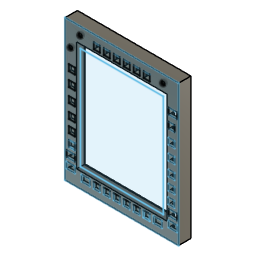
Portrait Iteration 4 v1 (Autodesk Fusion 360 design; units mm, degrees)
Autodesk Fusion 360 part; units mm, degrees
sketch "Sketch1" plane through (0, 0, 0) normal (0, 1, 0) x (1, 0, 0)
  line L0 (-16.7763, -52.2646) -> (91.3257, -52.2646)
  line L1 (91.3257, -52.2646) -> (91.3257, 81.2454)
  line L2 (91.3257, 81.2454) -> (-16.7763, 81.2454)
  line L3 (-16.7763, 81.2454) -> (-16.7763, -52.2646)
  line L4 (-36.7763, -77.2646) -> (111.3257, -77.2646)
  line L5 (111.3257, -77.2646) -> (111.3257, 106.2454)
  line L6 (111.3257, 106.2454) -> (-36.7763, 106.2454)
  line L7 (-36.7763, 106.2454) -> (-36.7763, -77.2646)
  dimension "d1" = 108.102
  dimension "d2" = 133.51
  dimension "d3" = 20
  dimension "d4" = 25
  dimension "d5" = 20
  dimension "d6" = 25
  constraint horizontal L0
  constraint vertical L1
  constraint horizontal L2
  constraint vertical L3
  constraint horizontal L4
  constraint vertical L5
  constraint horizontal L6
  constraint vertical L7
  measures "d1" distance of L0.start L0.end
  measures "d2" distance of L0.start L2.end
  measures "d3" distance of L1 L5
  measures "d4" distance of L2 L6
  measures "d5" distance of L3 L7
  measures "d6" distance of L0 L4
extrude "Extrude1" add sketch "Sketch1" along normal blind 16
chamfer "Chamfer1" distance 5 angle 45 4 edges at (-16.7763, 0, -14.4904) (37.2747, 0, 52.2646) (91.3257, 0, -14.4904) (37.2747, 0, -81.2454)
sketch "Sketch2" plane through (0, 0, 0) normal (0, -1, 0) x (1, 0, 0)
  line L0 (-36.7763, 77.2646) -> (-36.7763, -106.2454)
  line L1 (-36.7763, -106.2454) -> (111.3257, -106.2454)
  line L2 (111.3257, -106.2454) -> (111.3257, 77.2646)
  line L3 (111.3257, 77.2646) -> (-36.7763, 77.2646)
  line L4 (-21.7763, -86.2454) -> (-21.7763, 57.2646)
  line L5 (-21.7763, 57.2646) -> (96.3257, 57.2646)
  line L6 (96.3257, 57.2646) -> (96.3257, -86.2454)
  line L7 (96.3257, -86.2454) -> (-21.7763, -86.2454)
  line L8 (-31.7763, 27.2646) -> (-23.7763, 27.2646)
  line L9 (-23.7763, 27.2646) -> (-23.7763, 19.2646)
  line L10 (-23.7763, 19.2646) -> (-31.7763, 19.2646)
  line L11 (-31.7763, 19.2646) -> (-31.7763, 27.2646)
  line L12 (-31.7763, -8.7354) -> (-23.7763, -8.7354)
  line L13 (-23.7763, -8.7354) -> (-23.7763, -16.7354)
  line L14 (-23.7763, -16.7354) -> (-31.7763, -16.7354)
  line L15 (-31.7763, -16.7354) -> (-31.7763, -8.7354)
  line L16 (-31.7763, 9.2646) -> (-23.7763, 9.2646)
  line L17 (-23.7763, 9.2646) -> (-23.7763, 1.2646)
  line L18 (-23.7763, 1.2646) -> (-31.7763, 1.2646)
  line L19 (-31.7763, 1.2646) -> (-31.7763, 9.2646)
  line L20 (-31.7763, -26.7354) -> (-23.7763, -26.7354)
  line L21 (-23.7763, -26.7354) -> (-23.7763, -34.7354)
  line L22 (-23.7763, -34.7354) -> (-31.7763, -34.7354)
  line L23 (-31.7763, -34.7354) -> (-31.7763, -26.7354)
  line L24 (-31.7763, -42.7354) -> (-23.7763, -42.7354)
  line L25 (-23.7763, -42.7354) -> (-23.7763, -50.7354)
  line L26 (-23.7763, -50.7354) -> (-31.7763, -50.7354)
  line L27 (-31.7763, -50.7354) -> (-31.7763, -42.7354)
  line L28 (-31.7763, -58.2454) -> (-23.7763, -58.2454)
  line L29 (-23.7763, -58.2454) -> (-23.7763, -66.2454)
  line L30 (-23.7763, -66.2454) -> (-31.7763, -66.2454)
  line L31 (-31.7763, -66.2454) -> (-31.7763, -58.2454)
  line L32 (0.7237, 68.2646) -> (8.7237, 68.2646)
  line L33 (8.7237, 68.2646) -> (8.7237, 60.2646)
  line L34 (8.7237, 60.2646) -> (0.7237, 60.2646)
  line L35 (0.7237, 60.2646) -> (0.7237, 68.2646)
  line L36 (13.7237, 60.2646) -> (13.7237, 68.2646)
  line L37 (13.7237, 68.2646) -> (21.7237, 68.2646)
  line L38 (21.7237, 68.2646) -> (21.7237, 60.2646)
  line L39 (21.7237, 60.2646) -> (13.7237, 60.2646)
  line L40 (26.7237, 60.2646) -> (26.7237, 68.2646)
  line L41 (26.7237, 68.2646) -> (34.7237, 68.2646)
  line L42 (34.7237, 68.2646) -> (34.7237, 60.2646)
  line L43 (34.7237, 60.2646) -> (26.7237, 60.2646)
  line L44 (65.7237, 60.2646) -> (65.7237, 68.2646)
  line L45 (65.7237, 68.2646) -> (73.7237, 68.2646)
  line L46 (73.7237, 68.2646) -> (73.7237, 60.2646)
  line L47 (73.7237, 60.2646) -> (65.7237, 60.2646)
  line L48 (39.7237, 60.2646) -> (39.7237, 68.2646)
  line L49 (39.7237, 68.2646) -> (47.7237, 68.2646)
  line L50 (47.7237, 68.2646) -> (47.7237, 60.2646)
  line L51 (47.7237, 60.2646) -> (39.7237, 60.2646)
  line L52 (52.7237, 60.2646) -> (52.7237, 68.2646)
  line L53 (52.7237, 68.2646) -> (60.7237, 68.2646)
  line L54 (60.7237, 68.2646) -> (60.7237, 60.2646)
  line L55 (60.7237, 60.2646) -> (52.7237, 60.2646)
  line L56 (98.3257, 27.2646) -> (106.3257, 27.2646)
  line L57 (106.3257, 27.2646) -> (106.3257, 19.2646)
  line L58 (106.3257, 19.2646) -> (98.3257, 19.2646)
  line L59 (98.3257, 19.2646) -> (98.3257, 27.2646)
  line L60 (98.3257, 9.2646) -> (106.3257, 9.2646)
  line L61 (106.3257, 9.2646) -> (106.3257, 1.2646)
  line L62 (106.3257, 1.2646) -> (98.3257, 1.2646)
  line L63 (98.3257, 1.2646) -> (98.3257, 9.2646)
  line L64 (98.3257, -8.7354) -> (106.3257, -8.7354)
  line L65 (106.3257, -8.7354) -> (106.3257, -16.7354)
  line L66 (106.3257, -16.7354) -> (98.3257, -16.7354)
  line L67 (98.3257, -16.7354) -> (98.3257, -8.7354)
  line L68 (98.3257, -26.7354) -> (106.3257, -26.7354)
  line L69 (106.3257, -26.7354) -> (106.3257, -34.7354)
  line L70 (106.3257, -34.7354) -> (98.3257, -34.7354)
  line L71 (98.3257, -34.7354) -> (98.3257, -26.7354)
  line L72 (98.3257, -42.7354) -> (106.3257, -42.7354)
  line L73 (106.3257, -42.7354) -> (106.3257, -50.7354)
  line L74 (106.3257, -50.7354) -> (98.3257, -50.7354)
  line L75 (98.3257, -50.7354) -> (98.3257, -42.7354)
  line L76 (97.8961, -58.2454) -> (105.8961, -58.2454)
  line L77 (105.8961, -58.2454) -> (105.8961, -66.2454)
  line L78 (105.8961, -66.2454) -> (97.8961, -66.2454)
  line L79 (97.8961, -66.2454) -> (97.8961, -58.2454)
  line L80 (0.7237, -89.2454) -> (8.7237, -89.2454)
  line L81 (8.7237, -89.2454) -> (8.7237, -97.2454)
  line L82 (8.7237, -97.2454) -> (0.7237, -97.2454)
  line L83 (0.7237, -97.2454) -> (0.7237, -89.2454)
  line L84 (13.7237, -89.2454) -> (21.7237, -89.2454)
  line L85 (21.7237, -89.2454) -> (21.7237, -97.2454)
  line L86 (13.7237, -97.2454) -> (13.7237, -89.2454)
  line L87 (21.7237, -97.2454) -> (13.7237, -97.2454)
  line L88 (26.7237, -89.2454) -> (34.7237, -89.2454)
  line L89 (34.7237, -89.2454) -> (34.7237, -97.2454)
  line L90 (26.7237, -97.2454) -> (26.7237, -89.2454)
  line L91 (34.7237, -97.2454) -> (26.7237, -97.2454)
  line L92 (39.7237, -89.2454) -> (47.7237, -89.2454)
  line L93 (47.7237, -89.2454) -> (47.7237, -97.2454)
  line L94 (39.7237, -97.2454) -> (39.7237, -89.2454)
  line L95 (47.7237, -97.2454) -> (39.7237, -97.2454)
  line L96 (52.7237, -89.2454) -> (60.7237, -89.2454)
  line L97 (60.7237, -89.2454) -> (60.7237, -97.2454)
  line L98 (52.7237, -97.2454) -> (52.7237, -89.2454)
  line L99 (60.7237, -97.2454) -> (52.7237, -97.2454)
  line L100 (65.7237, -89.2454) -> (73.7237, -89.2454)
  line L101 (73.7237, -89.2454) -> (73.7237, -97.2454)
  line L102 (65.7237, -97.2454) -> (65.7237, -89.2454)
  line L103 (73.7237, -97.2454) -> (65.7237, -97.2454)
  line L104 (65.7237, -97.2454) -> (65.7237, -89.2454)
  line L105 (65.7237, -89.2454) -> (73.7237, -89.2454)
  line L106 (73.7237, -89.2454) -> (73.7237, -97.2454)
  line L107 (73.7237, -97.2454) -> (65.7237, -97.2454)
  line L108 (78.7237, -97.2454) -> (78.7237, -89.2454)
  line L109 (78.7237, -89.2454) -> (89.7237, -89.2454)
  line L110 (89.7237, -89.2454) -> (89.7237, -97.2454)
  line L111 (89.7237, -97.2454) -> (78.7237, -97.2454)
  line L112 (-15.2763, -89.2454) -> (-4.2763, -89.2454)
  line L113 (-4.2763, -89.2454) -> (-4.2763, -97.2454)
  line L114 (-4.2763, -97.2454) -> (-15.2763, -97.2454)
  line L115 (-15.2763, -97.2454) -> (-15.2763, -89.2454)
  line L116 (-31.7763, -58.2454) -> (-23.7763, -58.2454)
  line L117 (-23.7763, -58.2454) -> (-23.7763, -66.2454)
  line L118 (-23.7763, -66.2454) -> (-31.7763, -66.2454)
  line L119 (-31.7763, -66.2454) -> (-31.7763, -58.2454)
  line L120 (-34.7763, -71.2454) -> (-23.7763, -71.2454)
  line L121 (-23.7763, -71.2454) -> (-23.7763, -79.2454)
  line L122 (-23.7763, -79.2454) -> (-34.7763, -79.2454)
  line L123 (-34.7763, -79.2454) -> (-34.7763, -71.2454)
  line L124 (-34.7763, -84.2454) -> (-23.7763, -84.2454)
  line L125 (-23.7763, -84.2454) -> (-23.7763, -92.2454)
  line L126 (-23.7763, -92.2454) -> (-34.7763, -92.2454)
  line L127 (-34.7763, -92.2454) -> (-34.7763, -84.2454)
  line L128 (98.3257, 43.2646) -> (109.3257, 43.2646)
  line L129 (109.3257, 43.2646) -> (109.3257, 35.2646)
  line L130 (109.3257, 35.2646) -> (98.3257, 35.2646)
  line L131 (98.3257, 35.2646) -> (98.3257, 43.2646)
  line L132 (98.3257, -71.2454) -> (109.3257, -71.2454)
  line L133 (109.3257, -71.2454) -> (109.3257, -79.2454)
  line L134 (109.3257, -79.2454) -> (98.3257, -79.2454)
  line L135 (98.3257, -79.2454) -> (98.3257, -71.2454)
  line L136 (98.3257, -84.2454) -> (109.3257, -84.2454)
  line L137 (109.3257, -84.2454) -> (109.3257, -92.2454)
  line L138 (109.3257, -92.2454) -> (98.3257, -92.2454)
  line L139 (98.3257, -92.2454) -> (98.3257, -84.2454)
  circle A0 centre (-16.7763, 67.2646) radius 1.8
  circle A1 centre (91.3257, 67.2646) radius 1.8
  circle A2 centre (-29.2763, 47.2646) radius 1.8
  dimension "d10" = 8
  dimension "d11" = 8
  dimension "d12" = 8
  dimension "d13" = 8
  dimension "d14" = 8
  dimension "d15" = 8
  dimension "d16" = 8
  dimension "d17" = 8
  dimension "d18" = 8
  dimension "d19" = 8
  dimension "d20" = 8
  dimension "d21" = 8
  dimension "d22" = 8
  dimension "d24" = 8
  dimension "d26" = 8
  dimension "d28" = 8
  dimension "d30" = 8
  dimension "d32" = 8
  dimension "d34" = 148.102
  dimension "d35" = 50
  dimension "d36" = 2
  dimension "d37" = 2
  dimension "d38" = 68
  dimension "d39" = 86
  dimension "d40" = 2
  dimension "d41" = 2
  dimension "d42" = 2
  dimension "d43" = 2
  dimension "d44" = 104
  dimension "d45" = 120
  dimension "d47" = 3
  dimension "d48" = 3
  dimension "d49" = 3
  dimension "d50" = 3
  dimension "d51" = 3
  dimension "d52" = 3
  dimension "d53" = 37.5
  dimension "d54" = 50.5
  dimension "d57" = 76.5
  dimension "d58" = 89.5
  dimension "d59" = 63.5
  dimension "d60" = 102.5
  dimension "d61" = 5
  dimension "d62" = 5
  dimension "d63" = 5
  dimension "d64" = 5
  dimension "d65" = 5
  dimension "d66" = 37.602
  dimension "d67" = 37.5
  dimension "d70" = 8
  dimension "d71" = 10
  dimension "d73" = 8
  dimension "d74" = 8
  dimension "d75" = 2
  dimension "d76" = 8
  dimension "d77" = 8
  dimension "d78" = 8
  dimension "d79" = 8
  dimension "d80" = 8
  dimension "d81" = 8
  dimension "d82" = 8
  dimension "d83" = 8
  dimension "d84" = 8
  dimension "d85" = 8
  dimension "d86" = 8
  dimension "d87" = 8
  dimension "d88" = 8
  dimension "d89" = 8
  dimension "d90" = 8
  dimension "d91" = 8
  dimension "d92" = 8
  dimension "d93" = 5
  dimension "d94" = 5
  dimension "d95" = 5
  dimension "d96" = 5
  dimension "d97" = 5
  dimension "d98" = 3
  dimension "d99" = 3
  dimension "d100" = 3
  dimension "d101" = 8
  dimension "d102" = 8
  dimension "d103" = 3
  dimension "d104" = 3
  dimension "d105" = 3
  dimension "d106" = 8
  dimension "d107" = 11
  dimension "d108" = 5
  dimension "d109" = 11
  dimension "d110" = 5
  dimension "d111" = 8
  dimension "d112" = 8
  dimension "d113" = 11
  dimension "d114" = 8
  dimension "d115" = 2
  dimension "d116" = 5
  dimension "d117" = 11
  dimension "d118" = 8
  dimension "d119" = 5
  dimension "d120" = 11
  dimension "d121" = 8
  dimension "d122" = 2
  dimension "d123" = 8
  dimension "d124" = 11
  dimension "d125" = 8
  dimension "d126" = 11
  dimension "d127" = 5
  dimension "d128" = 2
  dimension "d129" = 11
  dimension "d130" = 8
  dimension "d131" = 11
  dimension "d132" = 5
  dimension "d133" = 3.6
  dimension "d134" = 10
  dimension "d135" = 20
  dimension "d136" = 37.5
  dimension "d137" = 20
  dimension "d138" = 3.6
  dimension "d139" = 10
  dimension "d140" = 20
  dimension "d141" = 3.6
  dimension "d142" = 5
  dimension "d143" = 7.5
  dimension "d144" = 7.5
  dimension "d145" = 30
  constraint horizontal L8
  constraint vertical L9
  constraint horizontal L10
  constraint vertical L11
  constraint horizontal L12
  constraint vertical L13
  constraint horizontal L14
  constraint vertical L15
  constraint horizontal L16
  constraint vertical L17
  constraint horizontal L18
  constraint vertical L19
  constraint horizontal L20
  constraint vertical L21
  constraint horizontal L22
  constraint vertical L23
  constraint horizontal L24
  constraint vertical L25
  constraint horizontal L26
  constraint vertical L27
  constraint horizontal L28
  constraint vertical L29
  constraint horizontal L30
  constraint vertical L31
  constraint horizontal L32
  constraint vertical L33
  constraint horizontal L34
  constraint vertical L35
  constraint horizontal L37
  constraint vertical L38
  constraint horizontal L39
  constraint vertical L36
  constraint horizontal L41
  constraint vertical L42
  constraint horizontal L43
  constraint vertical L40
  constraint horizontal L45
  constraint vertical L46
  constraint horizontal L47
  constraint vertical L44
  constraint horizontal L49
  constraint vertical L50
  constraint horizontal L51
  constraint vertical L48
  constraint horizontal L53
  constraint vertical L54
  constraint horizontal L55
  constraint vertical L52
  constraint horizontal L56
  constraint vertical L57
  constraint horizontal L58
  constraint vertical L59
  constraint horizontal L60
  constraint vertical L61
  constraint horizontal L62
  constraint vertical L63
  constraint horizontal L64
  constraint vertical L65
  constraint horizontal L66
  constraint vertical L67
  constraint horizontal L68
  constraint vertical L69
  constraint horizontal L70
  constraint vertical L71
  constraint horizontal L72
  constraint vertical L73
  constraint horizontal L74
  constraint vertical L75
  constraint horizontal L76
  constraint vertical L77
  constraint horizontal L78
  constraint vertical L79
  constraint horizontal L80
  constraint vertical L81
  constraint horizontal L82
  constraint vertical L83
  constraint horizontal L84
  constraint vertical L85
  constraint horizontal L87
  constraint vertical L86
  constraint horizontal L88
  constraint vertical L89
  constraint horizontal L91
  constraint vertical L90
  constraint horizontal L100
  constraint vertical L101
  constraint horizontal L103
  constraint vertical L102
  constraint horizontal L92
  constraint vertical L93
  constraint horizontal L95
  constraint vertical L94
  constraint horizontal L96
  constraint vertical L97
  constraint horizontal L99
  constraint vertical L98
  constraint horizontal L105
  constraint vertical L106
  constraint horizontal L107
  constraint vertical L104
  constraint horizontal L109
  constraint vertical L110
  constraint horizontal L111
  constraint vertical L108
  constraint horizontal L112
  constraint vertical L113
  constraint horizontal L114
  constraint vertical L115
  constraint horizontal L116
  constraint vertical L117
  constraint horizontal L118
  constraint vertical L119
  constraint horizontal L120
  constraint vertical L121
  constraint horizontal L122
  constraint vertical L123
  constraint horizontal L124
  constraint vertical L125
  constraint horizontal L126
  constraint vertical L127
  constraint horizontal L128
  constraint vertical L129
  constraint horizontal L130
  constraint vertical L131
  constraint horizontal L132
  constraint vertical L133
  constraint horizontal L134
  constraint vertical L135
  constraint horizontal L136
  constraint vertical L137
  constraint horizontal L138
  constraint vertical L139
  measures "d10" distance of L8.start L8.end
  measures "d11" distance of L8.start L10.end
  measures "d12" distance of L12.end L12.start
  measures "d13" distance of L14.end L12.start
  measures "d14" distance of L16.end L16.start
  measures "d15" distance of L18.end L16.start
  measures "d16" distance of L20.end L20.start
  measures "d17" distance of L22.end L20.start
  measures "d18" distance of L24.end L24.start
  measures "d19" distance of L26.end L24.start
  measures "d20" distance of L28.end L28.start
  measures "d21" distance of L30.end L28.start
  measures "d22" distance of L32.end L32.start
  measures "d24" distance of L37.end L36.end
  measures "d26" distance of L41.end L40.end
  measures "d28" distance of L45.end L44.end
  measures "d30" distance of L49.end L48.end
  measures "d32" distance of L53.end L52.end
  measures "d34" distance of L0.start L2.end
  measures "d35" distance of L3 L8
  measures "d36" distance of L4 L9
  measures "d37" distance of L4 L17
  measures "d38" distance of L3 L16
  measures "d39" distance of L3 L12
  measures "d40" distance of L4 L13
  measures "d41" distance of L4 L21
  measures "d42" distance of L4 L25
  measures "d43" distance of L4 L29
  measures "d44" distance of L3 L20
  measures "d45" distance of L3 L24
  measures "d47" distance of L5 L34
  measures "d48" distance of L5 L39
  measures "d49" distance of L5 L43
  measures "d50" distance of L5 L47
  measures "d51" distance of L5 L51
  measures "d52" distance of L5 L55
  measures "d53" distance of L0 L35
  measures "d54" distance of L0 L36
  measures "d57" distance of L0 L48
  measures "d58" distance of L0 L52
  measures "d59" distance of L0 L40
  measures "d60" distance of L0 L44
  measures "d61" distance of L33 L36
  measures "d62" distance of L38 L40
  measures "d63" distance of L42 L48
  measures "d64" distance of L50 L52
  measures "d65" distance of L44 L54
  measures "d66" distance of L2 L46
  measures "d67" distance of L0 L35
  measures "d70" distance of L16.end L16.start
  measures "d71" distance of L10 L16
  measures "d73" distance of L56.end L56.start
  measures "d74" distance of L58.end L56.start
  measures "d75" distance of L6 L59
  measures "d76" distance of L60.start L60.end
  measures "d77" distance of L60.start L62.end
  measures "d78" distance of L60.start L60.end
  measures "d79" distance of L64.start L64.end
  measures "d80" distance of L64.start L66.end
  measures "d81" distance of L68.end L68.start
  measures "d82" distance of L68.start L70.end
  measures "d83" distance of L72.end L72.start
  measures "d84" distance of L72.start L74.end
  measures "d85" distance of L76.start L76.end
  measures "d86" distance of L78.end L76.start
  measures "d87" distance of L80.end L80.start
  measures "d88" distance of L84.start L84.end
  measures "d89" distance of L88.start L88.end
  measures "d90" distance of L100.end L100.start
  measures "d91" distance of L92.start L92.end
  measures "d92" distance of L96.end L96.start
  measures "d93" distance of L81 L86
  measures "d94" distance of L85 L90
  measures "d95" distance of L89 L94
  measures "d96" distance of L93 L98
  measures "d97" distance of L97 L102
  measures "d98" distance of L7 L80
  measures "d99" distance of L7 L84
  measures "d100" distance of L7 L88
  measures "d101" distance of L92.start L92.end
  measures "d102" distance of L92.start L92.end
  measures "d103" distance of L7 L92
  measures "d104" distance of L7 L96
  measures "d105" distance of L7 L100
  measures "d106" distance of L100.end L100.start
  measures "d107" distance of L108.end L109.end
  measures "d108" distance of L106 L108
  measures "d109" distance of L112.start L112.end
  measures "d110" distance of L83 L113
  measures "d111" distance of L28.start L28.end
  measures "d112" distance of L30.end L28.start
  measures "d113" distance of L120.start L120.end
  measures "d114" distance of L120.start L122.end
  measures "d115" distance of L4 L121
  measures "d116" distance of L118 L120
  measures "d117" distance of L124.end L124.start
  measures "d118" distance of L126.end L124.start
  measures "d119" distance of L122 L124
  measures "d120" distance of L128.start L128.end
  measures "d121" distance of L128.start L130.end
  measures "d122" distance of L6 L131
  measures "d123" distance of L56 L130
  measures "d124" distance of L132.start L132.end
  measures "d125" distance of L132.start L134.end
  measures "d126" distance of L132.start L132.end
  measures "d127" distance of L78 L132
  measures "d128" distance of L6 L135
  measures "d129" distance of L136.end L136.start
  measures "d130" distance of L136.start L138.end
  measures "d131" distance of L136.end L136.start
  measures "d132" distance of L134 L136
  measures "d133" diameter of A0
  measures "d134" distance of L3 A0.centre
  measures "d135" distance of L3 L5
  measures "d136" distance of L0 L35
  measures "d137" distance of L0 A0.centre
  measures "d138" diameter of A1
  measures "d139" distance of L3 A1.centre
  measures "d140" distance of L2 A1.centre
  measures "d141" diameter of A2
  measures "d142" distance of L0 L11
  measures "d143" distance of L0 A2.centre
  measures "d144" distance of L4 A2.centre
  measures "d145" distance of L3 A2.centre
extrude "Extrude2" cut sketch "Sketch2" against normal through all contours L8 L9 L10 L11 | L12 L13 L14 L15 | L16 L17 L18 L19 | L20 L21 L22 L23 | L24 L25 L26 L27 | L28 L29 L30 L31 L116 L117 L118 L119 | L32 L33 L34 L35 | L36 L37 L38 L39 | L40 L41 L42 L43 | L44 L45 L46 L47 | L48 L49 L50 L51 | L52 L53 L54 L55 | L56 L57 L58 L59 | L60 L61 L62 L63 | L64 L65 L66 L67 | L68 L69 L70 L71 | L72 L73 L74 L75 | L76 L77 L78 L79 | L80 L81 L82 L83 | L84 L85 L86 L87 | L88 L89 L90 L91 | L92 L93 L94 L95 | L96 L97 L98 L99 | L100 L101 L102 L103 L104 L105 L106 L107 | L108 L109 L110 L111 | L112 L113 L114 L115 | L120 L121 L122 L123 | L124 L125 L126 L127 | L128 L129 L130 L131 | L132 L133 L134 L135 | L136 L137 L138 L139 | A0 | A2
extrude "Extrude3" cut sketch "Sketch2" against normal through all contours A1
sketch "Sketch3" plane through (0, 16, 0) normal (0, 1, 0) x (-1, 0, 0)
  circle A0 centre (-91.3257, 67.2646) radius 1.8
  line L0 (34.7763, -71.2454) -> (34.7763, -79.2454)
  line L1 (34.7763, -79.2454) -> (23.7763, -79.2454)
  line L2 (23.7763, -79.2454) -> (23.7763, -71.2454)
  line L3 (23.7763, -71.2454) -> (34.7763, -71.2454)
  line L4 (-13.7237, -97.2454) -> (-21.7237, -97.2454)
  line L5 (-21.7237, -97.2454) -> (-21.7237, -89.2454)
  line L6 (-21.7237, -89.2454) -> (-13.7237, -89.2454)
  line L7 (-13.7237, -89.2454) -> (-13.7237, -97.2454)
  line L8 (-65.7237, -97.2454) -> (-73.7237, -97.2454)
  line L9 (-73.7237, -97.2454) -> (-73.7237, -89.2454)
  line L10 (-73.7237, -89.2454) -> (-65.7237, -89.2454)
  line L11 (-65.7237, -89.2454) -> (-65.7237, -97.2454)
  line L12 (-97.8961, -58.2454) -> (-97.8961, -66.2454)
  line L13 (-97.8961, -66.2454) -> (-105.8961, -66.2454)
  line L14 (-105.8961, -66.2454) -> (-105.8961, -58.2454)
  line L15 (-105.8961, -58.2454) -> (-97.8961, -58.2454)
  line L16 (-98.3257, 9.2646) -> (-98.3257, 1.2646)
  line L17 (-98.3257, 1.2646) -> (-106.3257, 1.2646)
  line L18 (-106.3257, 1.2646) -> (-106.3257, 9.2646)
  line L19 (-106.3257, 9.2646) -> (-98.3257, 9.2646)
  line L20 (-52.7237, 60.2646) -> (-60.7237, 60.2646)
  line L21 (-60.7237, 60.2646) -> (-60.7237, 68.2646)
  line L22 (-60.7237, 68.2646) -> (-52.7237, 68.2646)
  line L23 (-52.7237, 68.2646) -> (-52.7237, 60.2646)
  line L24 (-0.7237, 68.2646) -> (-0.7237, 60.2646)
  line L25 (-0.7237, 60.2646) -> (-8.7237, 60.2646)
  line L26 (-8.7237, 60.2646) -> (-8.7237, 68.2646)
  line L27 (-8.7237, 68.2646) -> (-0.7237, 68.2646)
  line L28 (31.7763, -8.7354) -> (31.7763, -16.7354)
  line L29 (31.7763, -16.7354) -> (23.7763, -16.7354)
  line L30 (23.7763, -16.7354) -> (23.7763, -8.7354)
  line L31 (23.7763, -8.7354) -> (31.7763, -8.7354)
  line L32 (31.7763, 9.2646) -> (31.7763, 1.2646)
  line L33 (31.7763, 1.2646) -> (23.7763, 1.2646)
  line L34 (23.7763, 1.2646) -> (23.7763, 9.2646)
  line L35 (23.7763, 9.2646) -> (31.7763, 9.2646)
  circle A1 centre (16.7763, 67.2646) radius 1.8
  line L36 (-39.7237, 60.2646) -> (-47.7237, 60.2646)
  line L37 (-47.7237, 60.2646) -> (-47.7237, 68.2646)
  line L38 (-47.7237, 68.2646) -> (-39.7237, 68.2646)
  line L39 (-39.7237, 68.2646) -> (-39.7237, 60.2646)
  line L40 (-98.3257, 27.2646) -> (-98.3257, 19.2646)
  line L41 (-98.3257, 19.2646) -> (-106.3257, 19.2646)
  line L42 (-106.3257, 19.2646) -> (-106.3257, 27.2646)
  line L43 (-106.3257, 27.2646) -> (-98.3257, 27.2646)
  line L44 (-98.3257, -42.7354) -> (-98.3257, -50.7354)
  line L45 (-98.3257, -50.7354) -> (-106.3257, -50.7354)
  line L46 (-106.3257, -50.7354) -> (-106.3257, -42.7354)
  line L47 (-106.3257, -42.7354) -> (-98.3257, -42.7354)
  line L48 (-78.7237, -97.2454) -> (-89.7237, -97.2454)
  line L49 (-89.7237, -97.2454) -> (-89.7237, -89.2454)
  line L50 (-89.7237, -89.2454) -> (-78.7237, -89.2454)
  line L51 (-78.7237, -89.2454) -> (-78.7237, -97.2454)
  line L52 (-26.7237, -97.2454) -> (-34.7237, -97.2454)
  line L53 (-34.7237, -97.2454) -> (-34.7237, -89.2454)
  line L54 (-34.7237, -89.2454) -> (-26.7237, -89.2454)
  line L55 (-26.7237, -89.2454) -> (-26.7237, -97.2454)
  line L56 (34.7763, -84.2454) -> (34.7763, -92.2454)
  line L57 (34.7763, -92.2454) -> (23.7763, -92.2454)
  line L58 (23.7763, -92.2454) -> (23.7763, -84.2454)
  line L59 (23.7763, -84.2454) -> (34.7763, -84.2454)
  line L60 (31.7763, -58.2454) -> (31.7763, -66.2454)
  line L61 (31.7763, -66.2454) -> (23.7763, -66.2454)
  line L62 (23.7763, -66.2454) -> (23.7763, -58.2454)
  line L63 (23.7763, -58.2454) -> (31.7763, -58.2454)
  line L64 (-0.7237, -89.2454) -> (-0.7237, -97.2454)
  line L65 (-0.7237, -97.2454) -> (-8.7237, -97.2454)
  line L66 (-8.7237, -97.2454) -> (-8.7237, -89.2454)
  line L67 (-8.7237, -89.2454) -> (-0.7237, -89.2454)
  line L68 (-52.7237, -97.2454) -> (-60.7237, -97.2454)
  line L69 (-60.7237, -97.2454) -> (-60.7237, -89.2454)
  line L70 (-60.7237, -89.2454) -> (-52.7237, -89.2454)
  line L71 (-52.7237, -89.2454) -> (-52.7237, -97.2454)
  line L72 (-98.3257, -71.2454) -> (-98.3257, -79.2454)
  line L73 (-98.3257, -79.2454) -> (-109.3257, -79.2454)
  line L74 (-109.3257, -79.2454) -> (-109.3257, -71.2454)
  line L75 (-109.3257, -71.2454) -> (-98.3257, -71.2454)
  line L76 (-98.3257, -8.7354) -> (-98.3257, -16.7354)
  line L77 (-98.3257, -16.7354) -> (-106.3257, -16.7354)
  line L78 (-106.3257, -16.7354) -> (-106.3257, -8.7354)
  line L79 (-106.3257, -8.7354) -> (-98.3257, -8.7354)
  line L80 (-65.7237, 60.2646) -> (-73.7237, 60.2646)
  line L81 (-73.7237, 60.2646) -> (-73.7237, 68.2646)
  line L82 (-73.7237, 68.2646) -> (-65.7237, 68.2646)
  line L83 (-65.7237, 68.2646) -> (-65.7237, 60.2646)
  line L84 (-13.7237, 60.2646) -> (-21.7237, 60.2646)
  line L85 (-21.7237, 60.2646) -> (-21.7237, 68.2646)
  line L86 (-21.7237, 68.2646) -> (-13.7237, 68.2646)
  line L87 (-13.7237, 68.2646) -> (-13.7237, 60.2646)
  line L88 (31.7763, -26.7354) -> (31.7763, -34.7354)
  line L89 (31.7763, -34.7354) -> (23.7763, -34.7354)
  line L90 (23.7763, -34.7354) -> (23.7763, -26.7354)
  line L91 (23.7763, -26.7354) -> (31.7763, -26.7354)
  line L92 (31.7763, 27.2646) -> (31.7763, 19.2646)
  line L93 (31.7763, 19.2646) -> (23.7763, 19.2646)
  line L94 (23.7763, 19.2646) -> (23.7763, 27.2646)
  line L95 (23.7763, 27.2646) -> (31.7763, 27.2646)
  circle A2 centre (29.2763, 47.2646) radius 1.8
  line L96 (-26.7237, 60.2646) -> (-34.7237, 60.2646)
  line L97 (-34.7237, 60.2646) -> (-34.7237, 68.2646)
  line L98 (-34.7237, 68.2646) -> (-26.7237, 68.2646)
  line L99 (-26.7237, 68.2646) -> (-26.7237, 60.2646)
  line L100 (-98.3257, 43.2646) -> (-98.3257, 35.2646)
  line L101 (-98.3257, 35.2646) -> (-109.3257, 35.2646)
  line L102 (-109.3257, 35.2646) -> (-109.3257, 43.2646)
  line L103 (-109.3257, 43.2646) -> (-98.3257, 43.2646)
  line L104 (-98.3257, -26.7354) -> (-98.3257, -34.7354)
  line L105 (-98.3257, -34.7354) -> (-106.3257, -34.7354)
  line L106 (-106.3257, -34.7354) -> (-106.3257, -26.7354)
  line L107 (-106.3257, -26.7354) -> (-98.3257, -26.7354)
  line L108 (-98.3257, -84.2454) -> (-98.3257, -92.2454)
  line L109 (-98.3257, -92.2454) -> (-109.3257, -92.2454)
  line L110 (-109.3257, -92.2454) -> (-109.3257, -84.2454)
  line L111 (-109.3257, -84.2454) -> (-98.3257, -84.2454)
  line L112 (-39.7237, -97.2454) -> (-47.7237, -97.2454)
  line L113 (-47.7237, -97.2454) -> (-47.7237, -89.2454)
  line L114 (-47.7237, -89.2454) -> (-39.7237, -89.2454)
  line L115 (-39.7237, -89.2454) -> (-39.7237, -97.2454)
  line L116 (15.2763, -89.2454) -> (15.2763, -97.2454)
  line L117 (15.2763, -97.2454) -> (4.2763, -97.2454)
  line L118 (4.2763, -97.2454) -> (4.2763, -89.2454)
  line L119 (4.2763, -89.2454) -> (15.2763, -89.2454)
  line L120 (31.7763, -42.7354) -> (31.7763, -50.7354)
  line L121 (31.7763, -50.7354) -> (23.7763, -50.7354)
  line L122 (23.7763, -50.7354) -> (23.7763, -42.7354)
  line L123 (23.7763, -42.7354) -> (31.7763, -42.7354)
  line L124 (16.7763, 52.2646) -> (16.7763, -81.2454)
  line L125 (16.7763, -81.2454) -> (-91.3257, -81.2454)
  line L126 (-91.3257, -81.2454) -> (-91.3257, 52.2646)
  line L127 (-91.3257, 52.2646) -> (16.7763, 52.2646)
  line L128 (36.7763, -106.2454) -> (36.7763, 77.2646)
  line L129 (36.7763, 77.2646) -> (-111.3257, 77.2646)
  line L130 (-111.3257, 77.2646) -> (-111.3257, -106.2454)
  line L131 (-111.3257, -106.2454) -> (36.7763, -106.2454)
  line L132 (-99.9567, 60.9686) -> (20.0433, 60.9686)
  line L133 (20.0433, 60.9686) -> (20.0433, -93.5314)
  line L134 (20.0433, -93.5314) -> (-99.9567, -93.5314)
  line L135 (-99.9567, -93.5314) -> (-99.9567, 60.9686)
  line L136 (16.7763, 52.2646) -> (-91.3257, 52.2646)
  line L137 (-91.3257, 52.2646) -> (-91.3257, -81.2454)
  line L138 (-91.3257, -81.2454) -> (16.7763, -81.2454)
  line L139 (16.7763, -81.2454) -> (16.7763, 52.2646)
  dimension "d148" = 120
  dimension "d149" = 154.5
  dimension "d150" = 8.704
  dimension "d151" = 8.631
  dimension "d152" = 12.286
  dimension "d153" = 3.267
  constraint horizontal L132
  constraint vertical L133
  constraint horizontal L134
  constraint vertical L135
  measures "d148" distance of L132.start L132.end
  measures "d149" distance of L132.end L133.end
  measures "d150" distance of L132 L136
  measures "d151" distance of L135 L137
  measures "d152" distance of L134 L138
  measures "d153" distance of L133 L139
extrude "Extrude4" cut sketch "Sketch3" against normal blind 10 contours L5 L6 L7 L9 L10 L11 L12 L13 L15 L16 L17 L19 L20 L21 L23 L24 L25 L26 L36 L37 L39 L40 L41 L43 L44 L45 L47 L49 L50 L51 L53 L54 L55 L64 L66 L67 L69 L70 L71 L72 L73 L75 L76 L77 L79 L80 L81 L83 L84 L85 L87 L96 L97 L99 L100 L101 L103 L104 L105 L107 L108 L109 L111 L113 L114 L115 L116 L118 L119 L132 L133 L134 L135
sketch "Sketch4" plane through (0, 16, 0) normal (0, 1, 0) x (-1, 0, 0)
  line L0 (-52.7237, 60.9686) -> (-47.7237, 60.9686)
  line L1 (-47.7237, 60.9686) -> (-47.7237, 68.2646)
  line L2 (-47.7237, 68.2646) -> (-39.7237, 68.2646)
  line L3 (-39.7237, 68.2646) -> (-39.7237, 60.9686)
  line L4 (-39.7237, 60.9686) -> (-34.7237, 60.9686)
  line L5 (-34.7237, 60.9686) -> (-34.7237, 68.2646)
  line L6 (-34.7237, 68.2646) -> (-26.7237, 68.2646)
  line L7 (-26.7237, 68.2646) -> (-26.7237, 60.9686)
  line L8 (-26.7237, 60.9686) -> (-21.7237, 60.9686)
  line L9 (-21.7237, 60.9686) -> (-21.7237, 68.2646)
  line L10 (-21.7237, 68.2646) -> (-13.7237, 68.2646)
  line L11 (-13.7237, 68.2646) -> (-13.7237, 60.9686)
  line L12 (-13.7237, 60.9686) -> (-8.7237, 60.9686)
  line L13 (-8.7237, 60.9686) -> (-8.7237, 68.2646)
  line L14 (-8.7237, 68.2646) -> (-0.7237, 68.2646)
  line L15 (-0.7237, 68.2646) -> (-0.7237, 60.9686)
  line L16 (-0.7237, 60.9686) -> (20.0433, 60.9686)
  line L17 (20.0433, 60.9686) -> (20.0433, -93.5314)
  line L18 (20.0433, -93.5314) -> (15.2763, -93.5314)
  line L19 (15.2763, -93.5314) -> (15.2763, -97.2454)
  line L20 (15.2763, -97.2454) -> (4.2763, -97.2454)
  line L21 (4.2763, -97.2454) -> (4.2763, -93.5314)
  line L22 (4.2763, -93.5314) -> (-0.7237, -93.5314)
  line L23 (-0.7237, -93.5314) -> (-0.7237, -97.2454)
  line L24 (-0.7237, -97.2454) -> (-8.7237, -97.2454)
  line L25 (-8.7237, -97.2454) -> (-8.7237, -93.5314)
  line L26 (-8.7237, -93.5314) -> (-13.7237, -93.5314)
  line L27 (-13.7237, -93.5314) -> (-13.7237, -97.2454)
  line L28 (-13.7237, -97.2454) -> (-21.7237, -97.2454)
  line L29 (-21.7237, -97.2454) -> (-21.7237, -93.5314)
  line L30 (-21.7237, -93.5314) -> (-26.7237, -93.5314)
  line L31 (-26.7237, -93.5314) -> (-26.7237, -97.2454)
  line L32 (-26.7237, -97.2454) -> (-34.7237, -97.2454)
  line L33 (-34.7237, -97.2454) -> (-34.7237, -93.5314)
  line L34 (-34.7237, -93.5314) -> (-39.7237, -93.5314)
  line L35 (-39.7237, -93.5314) -> (-39.7237, -97.2454)
  line L36 (-39.7237, -97.2454) -> (-47.7237, -97.2454)
  line L37 (-47.7237, -97.2454) -> (-47.7237, -93.5314)
  line L38 (-47.7237, -93.5314) -> (-52.7237, -93.5314)
  line L39 (-52.7237, -93.5314) -> (-52.7237, -97.2454)
  line L40 (-52.7237, -97.2454) -> (-60.7237, -97.2454)
  line L41 (-60.7237, -97.2454) -> (-60.7237, -93.5314)
  line L42 (-60.7237, -93.5314) -> (-65.7237, -93.5314)
  line L43 (-65.7237, -93.5314) -> (-65.7237, -97.2454)
  line L44 (-65.7237, -97.2454) -> (-73.7237, -97.2454)
  line L45 (-73.7237, -97.2454) -> (-73.7237, -93.5314)
  line L46 (-73.7237, -93.5314) -> (-78.7237, -93.5314)
  line L47 (-78.7237, -93.5314) -> (-78.7237, -97.2454)
  line L48 (-78.7237, -97.2454) -> (-89.7237, -97.2454)
  line L49 (-89.7237, -97.2454) -> (-89.7237, -93.5314)
  line L50 (-89.7237, -93.5314) -> (-99.9567, -93.5314)
  line L51 (-99.9567, -93.5314) -> (-99.9567, -92.2454)
  line L52 (-99.9567, -92.2454) -> (-109.3257, -92.2454)
  line L53 (-109.3257, -92.2454) -> (-109.3257, -84.2454)
  line L54 (-109.3257, -84.2454) -> (-99.9567, -84.2454)
  line L55 (-99.9567, -84.2454) -> (-99.9567, -79.2454)
  line L56 (-99.9567, -79.2454) -> (-109.3257, -79.2454)
  line L57 (-109.3257, -79.2454) -> (-109.3257, -71.2454)
  line L58 (-109.3257, -71.2454) -> (-99.9567, -71.2454)
  line L59 (-99.9567, -71.2454) -> (-99.9567, -66.2454)
  line L60 (-99.9567, -66.2454) -> (-105.8961, -66.2454)
  line L61 (-105.8961, -66.2454) -> (-105.8961, -58.2454)
  line L62 (-105.8961, -58.2454) -> (-99.9567, -58.2454)
  line L63 (-99.9567, -58.2454) -> (-99.9567, -50.7354)
  line L64 (-99.9567, -50.7354) -> (-106.3257, -50.7354)
  line L65 (-106.3257, -50.7354) -> (-106.3257, -42.7354)
  line L66 (-106.3257, -42.7354) -> (-99.9567, -42.7354)
  line L67 (-99.9567, -42.7354) -> (-99.9567, -34.7354)
  line L68 (-99.9567, -34.7354) -> (-106.3257, -34.7354)
  line L69 (-106.3257, -34.7354) -> (-106.3257, -26.7354)
  line L70 (-106.3257, -26.7354) -> (-99.9567, -26.7354)
  line L71 (-99.9567, -26.7354) -> (-99.9567, -16.7354)
  line L72 (-99.9567, -16.7354) -> (-106.3257, -16.7354)
  line L73 (-106.3257, -16.7354) -> (-106.3257, -8.7354)
  line L74 (-106.3257, -8.7354) -> (-99.9567, -8.7354)
  line L75 (-99.9567, -8.7354) -> (-99.9567, 1.2646)
  line L76 (-99.9567, 1.2646) -> (-106.3257, 1.2646)
  line L77 (-106.3257, 1.2646) -> (-106.3257, 9.2646)
  line L78 (-106.3257, 9.2646) -> (-99.9567, 9.2646)
  line L79 (-99.9567, 9.2646) -> (-99.9567, 19.2646)
  line L80 (-99.9567, 19.2646) -> (-106.3257, 19.2646)
  line L81 (-106.3257, 19.2646) -> (-106.3257, 27.2646)
  line L82 (-106.3257, 27.2646) -> (-99.9567, 27.2646)
  line L83 (-99.9567, 27.2646) -> (-99.9567, 35.2646)
  line L84 (-99.9567, 35.2646) -> (-109.3257, 35.2646)
  line L85 (-109.3257, 35.2646) -> (-109.3257, 43.2646)
  line L86 (-109.3257, 43.2646) -> (-99.9567, 43.2646)
  line L87 (-99.9567, 43.2646) -> (-99.9567, 60.9686)
  line L88 (-99.9567, 60.9686) -> (-73.7237, 60.9686)
  line L89 (-73.7237, 60.9686) -> (-73.7237, 68.2646)
  line L90 (-73.7237, 68.2646) -> (-65.7237, 68.2646)
  line L91 (-65.7237, 68.2646) -> (-65.7237, 60.9686)
  line L92 (-65.7237, 60.9686) -> (-60.7237, 60.9686)
  line L93 (-60.7237, 60.9686) -> (-60.7237, 68.2646)
  line L94 (-60.7237, 68.2646) -> (-52.7237, 68.2646)
  line L95 (-52.7237, 68.2646) -> (-52.7237, 60.9686)
  circle A0 centre (-91.3257, 67.2646) radius 1.8
  line L96 (34.7763, -71.2454) -> (34.7763, -79.2454)
  line L97 (34.7763, -79.2454) -> (23.7763, -79.2454)
  line L98 (23.7763, -79.2454) -> (23.7763, -71.2454)
  line L99 (23.7763, -71.2454) -> (34.7763, -71.2454)
  line L100 (31.7763, -8.7354) -> (31.7763, -16.7354)
  line L101 (31.7763, -16.7354) -> (23.7763, -16.7354)
  line L102 (23.7763, -16.7354) -> (23.7763, -8.7354)
  line L103 (23.7763, -8.7354) -> (31.7763, -8.7354)
  line L104 (31.7763, 9.2646) -> (31.7763, 1.2646)
  line L105 (31.7763, 1.2646) -> (23.7763, 1.2646)
  line L106 (23.7763, 1.2646) -> (23.7763, 9.2646)
  line L107 (23.7763, 9.2646) -> (31.7763, 9.2646)
  circle A1 centre (16.7763, 67.2646) radius 1.8
  line L108 (34.7763, -84.2454) -> (34.7763, -92.2454)
  line L109 (34.7763, -92.2454) -> (23.7763, -92.2454)
  line L110 (23.7763, -92.2454) -> (23.7763, -84.2454)
  line L111 (23.7763, -84.2454) -> (34.7763, -84.2454)
  line L112 (31.7763, -58.2454) -> (31.7763, -66.2454)
  line L113 (31.7763, -66.2454) -> (23.7763, -66.2454)
  line L114 (23.7763, -66.2454) -> (23.7763, -58.2454)
  line L115 (23.7763, -58.2454) -> (31.7763, -58.2454)
  line L116 (31.7763, -26.7354) -> (31.7763, -34.7354)
  line L117 (31.7763, -34.7354) -> (23.7763, -34.7354)
  line L118 (23.7763, -34.7354) -> (23.7763, -26.7354)
  line L119 (23.7763, -26.7354) -> (31.7763, -26.7354)
  line L120 (31.7763, 27.2646) -> (31.7763, 19.2646)
  line L121 (31.7763, 19.2646) -> (23.7763, 19.2646)
  line L122 (23.7763, 19.2646) -> (23.7763, 27.2646)
  line L123 (23.7763, 27.2646) -> (31.7763, 27.2646)
  circle A2 centre (29.2763, 47.2646) radius 1.8
  line L124 (31.7763, -42.7354) -> (31.7763, -50.7354)
  line L125 (31.7763, -50.7354) -> (23.7763, -50.7354)
  line L126 (23.7763, -50.7354) -> (23.7763, -42.7354)
  line L127 (23.7763, -42.7354) -> (31.7763, -42.7354)
  line L128 (36.7763, -106.2454) -> (36.7763, 77.2646)
  line L129 (36.7763, 77.2646) -> (-111.3257, 77.2646)
  line L130 (-111.3257, 77.2646) -> (-111.3257, -106.2454)
  line L131 (-111.3257, -106.2454) -> (36.7763, -106.2454)
  line L132 (-108.3257, 60.9686) -> (-99.9567, 60.9686)
  line L133 (-99.9567, 60.9686) -> (-99.9567, -92.565)
  line L134 (-99.9567, -92.565) -> (-108.3257, -92.565)
  line L135 (-108.3257, -92.565) -> (-108.3257, 60.9686)
  line L136 (-111.3257, 77.2646) -> (-111.3257, -106.2454)
  line L137 (-108.3257, 74.2646) -> (33.7763, 74.2646)
  line L138 (33.7763, 74.2646) -> (33.7763, 60.9686)
  line L139 (33.7763, 60.9686) -> (-108.3257, 60.9686)
  line L140 (-108.3257, 60.9686) -> (-108.3257, 74.2646)
  line L141 (36.7763, -106.2454) -> (36.7763, 77.2646)
  line L142 (36.7763, 77.2646) -> (-111.3257, 77.2646)
  line L143 (-108.3257, -100.1775) -> (33.7763, -100.1775)
  line L144 (33.7763, -100.1775) -> (33.7763, -92.565)
  line L145 (33.7763, -92.565) -> (-108.3257, -92.565)
  line L146 (-108.3257, -92.565) -> (-108.3257, -100.1775)
  line L147 (33.7763, 60.9686) -> (20.0433, 60.9686)
  line L148 (20.0433, 60.9686) -> (20.0433, -92.565)
  line L149 (20.0433, -92.565) -> (33.7763, -92.565)
  line L150 (33.7763, -92.565) -> (33.7763, 60.9686)
  dimension "d156" = 3
  dimension "d157" = 3
  dimension "d158" = 3
  dimension "d161" = 3
  dimension "d162" = 3
  dimension "d163" = 3
  dimension "d164" = 3
  constraint horizontal L132
  constraint vertical L133
  constraint horizontal L134
  constraint vertical L135
  constraint collinear L55 L133
  constraint horizontal L137
  constraint vertical L138
  constraint horizontal L139
  constraint vertical L140
  constraint collinear L88 L139
  constraint collinear L132 L139
  constraint horizontal L143
  constraint vertical L144
  constraint horizontal L145
  constraint vertical L146
  constraint collinear L134 L145
  constraint horizontal L147
  constraint vertical L148
  constraint horizontal L149
  constraint vertical L150
  constraint collinear L17 L148
  constraint collinear L145 L149
  constraint collinear L139 L147
  measures "d156" distance of L135 L136
  measures "d157" distance of L138 L141
  measures "d158" distance of L136 L140
  measures "d161" distance of L137 L142
  measures "d162" distance of L141 L144
  measures "d163" distance of L136 L146
  measures "d164" distance of L141 L150
extrude "Extrude5" cut sketch "Sketch4" against normal blind 13 contours L0 L1 L2 L3 L4 L5 L6 L7 L8 L9 L10 L11 L12 L13 L14 L15 L16 L88 L89 L90 L91 L92 L93 L94 L95 L132 L137 L138 L139 L140 L147 | L86 L87 L132 L133 L135 L139 | L58 L59 L60 L61 L62 L63 L64 L65 L66 L67 L68 L69 L70 L71 L72 L73 L74 L75 L76 L77 L78 L79 L80 L81 L82 L83 L84 L133 L135 | L17 L97 L98 L99 L109 L110 L111 L139 L145 L147 L148 L149 L150 | L54 L55 L56 L133 L135 | L17 L18 L19 L20 L21 L22 L23 L24 L25 L26 L27 L28 L29 L30 L31 L32 L33 L34 L35 L36 L37 L38 L39 L40 L41 L42 L43 L44 L45 L46 L47 L48 L49 L50 L51 L134 L143 L144 L145 L146 L149
sketch "Sketch5" plane through (0, 16, 0) normal (0, 1, 0) x (-1, 0, 0)
  line L0 (-108.3257, -84.2454) -> (-108.3257, -79.2454)
  line L1 (-108.3257, -79.2454) -> (-109.3257, -79.2454)
  line L2 (-109.3257, -79.2454) -> (-109.3257, -71.2454)
  line L3 (-109.3257, -71.2454) -> (-108.3257, -71.2454)
  line L4 (-108.3257, -71.2454) -> (-108.3257, 35.2646)
  line L5 (-108.3257, 35.2646) -> (-109.3257, 35.2646)
  line L6 (-109.3257, 35.2646) -> (-109.3257, 43.2646)
  line L7 (-109.3257, 43.2646) -> (-108.3257, 43.2646)
  line L8 (-108.3257, 43.2646) -> (-108.3257, 74.2646)
  line L9 (-108.3257, 74.2646) -> (33.7763, 74.2646)
  line L10 (33.7763, 74.2646) -> (33.7763, -71.2454)
  line L11 (33.7763, -71.2454) -> (34.7763, -71.2454)
  line L12 (34.7763, -71.2454) -> (34.7763, -79.2454)
  line L13 (34.7763, -79.2454) -> (33.7763, -79.2454)
  line L14 (33.7763, -79.2454) -> (33.7763, -84.2454)
  line L15 (33.7763, -84.2454) -> (34.7763, -84.2454)
  line L16 (34.7763, -84.2454) -> (34.7763, -92.2454)
  line L17 (34.7763, -92.2454) -> (33.7763, -92.2454)
  line L18 (33.7763, -92.2454) -> (33.7763, -100.1775)
  line L19 (33.7763, -100.1775) -> (-108.3257, -100.1775)
  line L20 (-108.3257, -100.1775) -> (-108.3257, -92.565)
  line L21 (-108.3257, -92.565) -> (-99.9567, -92.565)
  line L22 (-99.9567, -92.565) -> (-99.9567, -92.2454)
  line L23 (-99.9567, -92.2454) -> (-109.3257, -92.2454)
  line L24 (-109.3257, -92.2454) -> (-109.3257, -84.2454)
  line L25 (-109.3257, -84.2454) -> (-108.3257, -84.2454)
  line L26 (36.7763, -106.2454) -> (36.7763, 77.2646)
  line L27 (36.7763, 77.2646) -> (-111.3257, 77.2646)
  line L28 (-111.3257, 77.2646) -> (-111.3257, -106.2454)
  line L29 (-111.3257, -106.2454) -> (36.7763, -106.2454)
  line L30 (-108.3257, -92.565) -> (-108.3257, -92.2454)
  constraint coincident L20.end L21.start
  constraint coincident L23 L30.end
  constraint perpendicular L23 L30
extrude "Extrude6" cut sketch "Sketch5" against normal blind 13 contours L21 L22 L23 L30
